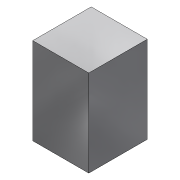
# Autodesk Inventor part: BLANK-BC-10005
Saved by Autodesk Inventor 2016 (Build 200138000, 138)
## iProperties
Created: 2015-12-02
Part Number: BLANK-BC-10005
Project: DIPOLO BC-3T- SIRIUS
Cost Center: 1504002005
Material: Aço Liga
Document SubType Name: Modeling
Designer: reinaldo.basilio.
Density: 8.08 g/cm^3
Appearance: Silver
Mass: 22179.6 g
Surface Area: 1196.7 cm^2
Volume: 2745 cm^3
Description: Polo do dipolo de 3 tesla.
RuleStatus: InUse
AfterMaterialChange0: file://_iMaterial
AfterAnyiPropertyChange0: file://_iMaterial
AfterDocNew0: file://_Naming_par
AfterDocNew1: file://_NameStart
AfterDocNew2: file://_NameStart1
AfterDocNew3: file://_Materiais
DocNumber: XXXXX-XXX-XXXX-00-001.ipt
Folder: .
Title: DIPOLO BC-3T- SIRIUS
Author: reinaldo.basilio
Subject: BLANK-BC-10005
Autodesk Inventor part; units mm, degrees
ref_plane "YZ Plane" through (0, 0, 0) normal (1, 0, 0) x (0, 1, 0)
ref_plane "XZ Plane" through (0, 0, 0) normal (0, 1, 0) x (-1, 0, 0)
ref_plane "XY Plane" through (0, 0, 0) normal (0, 0, 1) x (1, 0, 0)
sketch "Sketch7" plane through (0, 0, 0) normal (0, 0, 1) x (1, 0, 0)
  line L0 (60, -57.5) -> (-60, -57.5)
  line L1 (-60, -57.5) -> (-60, 57.5)
  line L2 (-60, 57.5) -> (60, 57.5)
  line L3 (60, 57.5) -> (60, -57.5)
  point P0 (0, 0)
  point P1 (0, -57.5)
  point P2 (-60, 0)
  dimension "d16" = 120
  dimension "d17" = 115
  constraints: 8 end point, 2 midpoint, 2 parallel, 1 horizontal, 1 horizontal alignment, 1 perpendicular, 1 vertical alignment
  measures "d16" distance of L1.end L2.end
  measures "d17" distance of L0.end L1.end
extrude "Extrusion7" add sketch "Sketch7" along normal blind 178
body "Solid6"
